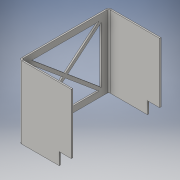
# Autodesk Inventor part: BatteryHolder
Saved by Autodesk Inventor 2016 (Build 200138000, 138)
## iProperties
Created: 2017-01-28
Part Number: BatteryHolder
Material: Generic
Document SubType Name: Sheet Metal
Designer: hamblettk
Density: 1 g/cm^3
Sheet Metal Rule: Default
Appearance: Default
Author: hamblettk
Autodesk Inventor part; units mm, degrees
ref_plane "YZ Plane" through (0, 0, 0) normal (1, 0, 0) x (0, 1, 0)
ref_plane "XZ Plane" through (0, 0, 0) normal (0, 1, 0) x (-1, 0, 0)
ref_plane "XY Plane" through (0, 0, 0) normal (0, 0, 1) x (1, 0, 0)
sketch "Sketch1" plane through (0, 0, 0) normal (1, 0, 0) x (0, 1, 0)
  line L0 (0, 0) -> (152.4, 0)
  line L1 (152.4, 0) -> (152.4, -336.55)
  line L2 (152.4, -336.55) -> (0, -336.55)
  line L3 (0, -336.55) -> (0, 0)
  dimension "d0" = 152.4
  dimension "d1" = 336.55
  measures "d0" distance of L1.end L2.end
  measures "d1" distance of L0.end L1.end
extrude "Plate1" add sketch "Sketch1" along normal blind 3.048
sketch "Sketch2" plane through (3.048, 0, 0) normal (1, 0, 0) x (0, 0, -1)
  line L0 (0, 152.4) -> (336.55, 152.4) projected
  line L1 (76.2, 152.4) -> (76.2, 0)
  line L2 (0, 0) -> (0, 152.4) projected
  dimension "d3" = 76.2
  constraints: 2 end point, 1 point on line, 1 vertical
  measures "d3" distance between parallel lines of L2 L1
fold "Fold1" angle 90 bend radius 3.048 thickness 3.048 k factor 0.44 line from (3.048, 152.4, -76.2) to (3.048, 0, -76.2) line at bend centre moving side (0, 0, 1) folds toward (1, 0, 0)
sketch "Sketch3" plane through (3.048, 0, 0) normal (1, 0, 0) x (0, 0, -1)
  line L0 (79.6472, 152.4) -> (336.55, 152.4) projected
  line L1 (260.35, 152.4) -> (260.35, 0)
  line L2 (336.55, 0) -> (79.6472, 0) projected
  line L3 (336.55, 152.4) -> (336.55, 0) projected
  point P0 (0, 0)
  dimension "d10" = 76.2
  constraints: 2 end point, 2 point on line, 1 vertical
  measures "d10" distance between parallel lines of L3 L1
fold "Fold2" angle 90 bend radius 3.048 thickness 3.048 k factor 0.44 line from (3.048, 152.4, -260.35) to (3.048, 0, -260.35) line at bend centre moving side (0, 0, -1) folds toward (1, 0, 0)
sketch "Sketch4" plane through (6.096, 0, -73.5512) normal (0, 0, 1) x (1, 0, 0)
  line L0 (72.7528, 0) -> (0, 0) projected
  line L1 (72.7528, 0) -> (47.0988, 0)
  line L2 (47.0988, 0) -> (47.0988, 25.654)
  line L3 (47.0988, 25.654) -> (72.7528, 25.654)
  line L4 (72.7528, 25.654) -> (72.7528, 0)
  point P0 (-6.096, 0)
  dimension "d17" = 25.654
  dimension "d18" = 25.654
  constraints: 8 end point, 2 parallel, 1 horizontal, 1 perpendicular
  measures "d17" distance of L2.end L3.end
  measures "d18" distance of L1.end L2.end
extrude "Extrusion1" cut sketch "Sketch4" against normal blind 336.55
sketch "Sketch5" plane through (0, 0, 0) normal (-1, 0, 0) x (0, 0, 1)
  line L0 (-79.6472, 0) -> (-79.6472, 152.4) projected
  line L1 (-79.6472, 152.4) -> (-256.9028, 152.4) projected
  line L2 (-256.9028, 152.4) -> (-256.9028, 0) projected
  line L3 (-256.9028, 0) -> (-79.6472, 0) projected
  line L4 (-244.2028, 16.839) -> (-173.2241, 76.2)
  line L5 (-239.2537, 12.7) -> (-168.275, 72.061)
  line L6 (-92.3472, 135.561) -> (-163.3259, 76.2)
  line L7 (-97.2963, 139.7) -> (-168.275, 80.339)
  line L8 (-239.2537, 139.7) -> (-168.275, 80.339)
  line L9 (-163.3259, 76.2) -> (-92.3472, 16.839)
  line L10 (-92.3472, 16.839) -> (-92.3472, 12.7)
  line L11 (-92.3472, 12.7) -> (-97.2963, 12.7)
  line L12 (-97.2963, 12.7) -> (-168.275, 72.061)
  line L13 (-173.2241, 76.2) -> (-244.2028, 135.561)
  line L14 (-244.2028, 135.561) -> (-244.2028, 139.7)
  line L15 (-239.2537, 139.7) -> (-244.2028, 139.7)
  line L16 (-244.2028, 16.839) -> (-244.2028, 12.7)
  line L17 (-244.2028, 12.7) -> (-239.2537, 12.7)
  line L18 (-92.3472, 135.561) -> (-92.3472, 139.7)
  line L19 (-97.2963, 139.7) -> (-92.3472, 139.7)
  line L20 (-244.2028, 139.7) -> (-92.3472, 139.7)
  line L21 (-92.3472, 139.7) -> (-92.3472, 12.7)
  line L22 (-92.3472, 12.7) -> (-244.2028, 12.7)
  line L23 (-244.2028, 12.7) -> (-244.2028, 139.7)
  point P0 (0, 0)
  constraints: 40 end point, 7 equal length, 6 point on line, 2 horizontal, 1 perpendicular
extrude "Extrusion2" cut sketch "Sketch5" against normal blind 3.175 contours L23 L13 L4 | L5 L12 L22 | L20 L7 L8 | L9 L6 L21
sketch "Sketch6" plane through (78.8488, 152.4, -73.5512) normal (1, 0, 0) x (0, 0, -1)
  line L0 (0, -126.746) -> (3.048, -126.746) projected
  line L1 (3.048, -126.746) -> (3.048, 0) projected
  line L2 (0, 0) -> (3.048, 0) projected
  line L3 (0, -126.746) -> (0, 0) projected
  line L4 (186.3996, -126.746) -> (189.4476, -126.746) projected
  line L5 (189.4476, 0) -> (189.4476, -126.746) projected
  line L6 (189.4476, 0) -> (186.3996, 0) projected
  line L7 (186.3996, 0) -> (186.3996, -126.746) projected
  point P0 (-73.5512, -152.4)
extrude "Extrusion3" add sketch "Sketch6" along normal blind 25.4
sketch "Sketch7" plane through (104.2488, 152.4, -73.5512) normal (1, 0, 0) x (0, 0, -1)
  line L0 (0, -126.746) -> (3.048, -126.746) projected
  line L1 (3.048, -126.746) -> (3.048, 0) projected
  line L2 (3.048, 0) -> (0, 0) projected
  line L3 (0, 0) -> (0, -126.746) projected
  line L4 (186.3996, -126.746) -> (189.4476, -126.746) projected
  line L5 (189.4476, -126.746) -> (189.4476, 0) projected
  line L6 (189.4476, 0) -> (186.3996, 0) projected
  line L7 (186.3996, 0) -> (186.3996, -126.746) projected
  point P0 (-73.5512, -152.4)
extrude "Extrusion4" add sketch "Sketch7" along normal blind 6.35
sketch "Sketch8" plane through (53.1948, 0, -73.5512) normal (1, 0, 0) x (0, 0, -1)
  line L0 (3.048, 25.654) -> (3.048, 0) projected
  line L1 (0, 25.654) -> (3.048, 25.654) projected
  line L2 (0, 0) -> (0, 25.654) projected
  line L3 (3.048, 0) -> (0, 0) projected
  line L4 (189.4476, 25.654) -> (189.4476, 0) projected
  line L5 (186.3996, 0) -> (186.3996, 25.654) projected
  line L6 (189.4476, 0) -> (186.3996, 0) projected
  line L7 (189.4476, 25.654) -> (189.4476, 0) projected
  line L8 (186.3996, 25.654) -> (189.4476, 25.654) projected
  point P0 (-73.5512, 0)
extrude "Extrusion5" add sketch "Sketch8" along normal blind 31.75
equation "\"d4\" = BendReliefWidth"
equation "\"d5\" = BendReliefDepth"
equation "\"d6\" = MinimumRemnant"
equation "\"d7\" = BendRadius"
equation "\"d9\" = BendRadius"
equation "\"d11\" = BendReliefWidth"
equation "\"d12\" = BendReliefDepth"
equation "\"d13\" = MinimumRemnant"
equation "\"d14\" = BendRadius"
equation "\"d16\" = BendRadius"
equation "\"BendRadius\" = Thickness"
equation "\"BendReliefWidth\" = Thickness"
equation "\"BendReliefDepth\" = 0.5 * Thickness"
equation "\"CornerReliefSize\" = 4 * Thickness"
equation "\"MinimumRemnant\" = 2 * Thickness"
equation "\"TransitionRadius\" = BendRadius"
equation "\"JacobiRadiusSize\" = BendRadius"
equation "\"GapSize\" = Thickness"
equation "\"d2\" = BendRadius"
equation "\"Thickness\" = 3.048"
body "Solid1"
